Autodesk Inventor part; units mm, degrees
(part 3 of 3)
  arc A665 (615.7426, 1908.5354) -> (603.7426, 1896.5354) centre (615.7426, 1896.5354) ccw
  line L665 (643.2426, 1896.5354) -> (643.2426, 1908.5354)
  line L666 (36.3541, 1810.6764) -> (36.3541, 1843.6764)
  line L667 (311.3541, 1810.6764) -> (311.3541, 1843.6764)
  line L668 (311.3541, 1810.6764) -> (36.3541, 1810.6764)
  circle A666 centre (233.6541, 1827.1764) radius 3
  circle A667 centre (114.0541, 1827.1764) radius 3
  line L669 (36.3541, 1843.6764) -> (36.3541, 1855.6764)
  line L670 (311.3541, 1855.6764) -> (36.3541, 1855.6764)
  line L671 (311.3541, 1843.6764) -> (311.3541, 1855.6764)
  line L672 (594.2448, 1855.6764) -> (594.2448, 1843.6764)
  line L673 (319.2448, 1855.6764) -> (319.2448, 1843.6764)
  line L674 (319.2448, 1855.6764) -> (594.2448, 1855.6764)
  line L675 (594.2448, 1810.6764) -> (594.2448, 1843.6764)
  line L676 (319.2448, 1810.6764) -> (594.2448, 1810.6764)
  line L677 (319.2448, 1810.6764) -> (319.2448, 1843.6764)
  circle A668 centre (516.5448, 1827.1764) radius 3
  circle A669 centre (396.9448, 1827.1764) radius 3
  line L678 (791.8708, 1824.2966) -> (651.8708, 1824.2966)
  arc A670 (791.8708, 1824.2966) -> (801.8708, 1834.2966) centre (791.8708, 1834.2966) ccw
  line L679 (801.8708, 1834.2966) -> (801.8708, 1845.2966)
  line L680 (841.3708, 1845.2966) -> (841.3708, 1812.2966)
  line L681 (841.3708, 1812.2966) -> (602.3708, 1812.2966)
  line L682 (602.3708, 1845.2966) -> (602.3708, 1812.2966)
  arc A671 (641.8708, 1834.2966) -> (651.8708, 1824.2966) centre (651.8708, 1834.2966) ccw
  line L683 (641.8708, 1834.2966) -> (641.8708, 1845.2966)
  line L684 (829.3708, 1857.2966) -> (801.8708, 1857.2966)
  arc A672 (841.3708, 1845.2966) -> (829.3708, 1857.2966) centre (829.3708, 1845.2966) ccw
  line L685 (801.8708, 1845.2966) -> (801.8708, 1857.2966)
  line L686 (641.8708, 1857.2966) -> (614.3708, 1857.2966)
  arc A673 (614.3708, 1857.2966) -> (602.3708, 1845.2966) centre (614.3708, 1845.2966) ccw
  line L687 (641.8708, 1845.2966) -> (641.8708, 1857.2966)
  line L688 (312.2332, 1586.4479) -> (37.2332, 1586.4479)
  line L689 (312.2332, 1586.4479) -> (312.2332, 1801.4479)
  line L690 (37.2332, 1801.4479) -> (37.2332, 1586.4479)
  line L691 (312.2332, 1801.4479) -> (37.2332, 1801.4479)
  line L692 (594.0537, 1587.8293) -> (319.0537, 1587.8293)
  line L693 (594.0537, 1587.8293) -> (594.0537, 1802.8293)
  line L694 (319.0537, 1802.8293) -> (319.0537, 1587.8293)
  line L695 (594.0537, 1802.8293) -> (319.0537, 1802.8293)
  line L696 (879.1815, 1586.5894) -> (604.1815, 1586.5894)
  line L697 (879.1815, 1586.5894) -> (879.1815, 1801.5894)
  line L698 (604.1815, 1801.5894) -> (604.1815, 1586.5894)
  line L699 (879.1815, 1801.5894) -> (604.1815, 1801.5894)
  line L700 (35.4953, 1536.4526) -> (274.4953, 1536.4526)
  line L701 (35.4953, 1569.4526) -> (35.4953, 1536.4526)
  line L702 (274.4953, 1569.4526) -> (274.4953, 1536.4526)
  line L703 (47.4953, 1581.4526) -> (262.4953, 1581.4526)
  arc A674 (274.4953, 1569.4526) -> (262.4953, 1581.4526) centre (262.4953, 1569.4526) ccw
  arc A675 (47.4953, 1581.4526) -> (35.4953, 1569.4526) centre (47.4953, 1569.4526) ccw
  line L704 (280.016, 1536.4526) -> (519.016, 1536.4526)
  line L705 (280.016, 1569.4526) -> (280.016, 1536.4526)
  line L706 (519.016, 1569.4526) -> (519.016, 1536.4526)
  line L707 (292.016, 1581.4526) -> (507.016, 1581.4526)
  arc A676 (519.016, 1569.4526) -> (507.016, 1581.4526) centre (507.016, 1569.4526) ccw
  arc A677 (292.016, 1581.4526) -> (280.016, 1569.4526) centre (292.016, 1569.4526) ccw
  line L708 (523.243, 1536.8823) -> (762.243, 1536.8823)
  line L709 (523.243, 1569.8823) -> (523.243, 1536.8823)
  line L710 (762.243, 1569.8823) -> (762.243, 1536.8823)
  line L711 (535.243, 1581.8823) -> (750.243, 1581.8823)
  arc A678 (762.243, 1569.8823) -> (750.243, 1581.8823) centre (750.243, 1569.8823) ccw
  arc A679 (535.243, 1581.8823) -> (523.243, 1569.8823) centre (535.243, 1569.8823) ccw
  circle A680 centre (711.5153, 1953.9544) radius 3
  circle A681 centre (651.7153, 1953.9544) radius 3
  arc A682 (711.5153, 1948.9544) -> (711.5153, 1958.9544) centre (711.5153, 1953.9544) ccw
  line L712 (711.5153, 1948.9544) -> (651.7153, 1948.9544)
  arc A683 (651.7153, 1958.9544) -> (651.7153, 1948.9544) centre (651.7153, 1953.9544) ccw
  line L713 (711.5153, 1958.9544) -> (651.7153, 1958.9544)
  circle A684 centre (786.612, 1954.088) radius 3
  circle A685 centre (726.812, 1954.088) radius 3
  arc A686 (786.612, 1949.088) -> (786.612, 1959.088) centre (786.612, 1954.088) ccw
  line L714 (786.612, 1949.088) -> (726.812, 1949.088)
  arc A687 (726.812, 1959.088) -> (726.812, 1949.088) centre (726.812, 1954.088) ccw
  line L715 (786.612, 1959.088) -> (726.812, 1959.088)
  circle A688 centre (711.8432, 1938.9091) radius 3
  circle A689 centre (652.0432, 1938.9091) radius 3
  arc A690 (711.8432, 1933.9091) -> (711.8432, 1943.9091) centre (711.8432, 1938.9091) ccw
  line L716 (711.8432, 1933.9091) -> (652.0432, 1933.9091)
  arc A691 (652.0432, 1943.9091) -> (652.0432, 1933.9091) centre (652.0432, 1938.9091) ccw
  line L717 (711.8432, 1943.9091) -> (652.0432, 1943.9091)
  circle A692 centre (786.9399, 1939.0427) radius 3
  circle A693 centre (727.1399, 1939.0427) radius 3
  arc A694 (786.9399, 1934.0427) -> (786.9399, 1944.0427) centre (786.9399, 1939.0427) ccw
  line L718 (786.9399, 1934.0427) -> (727.1399, 1934.0427)
  arc A695 (727.1399, 1944.0427) -> (727.1399, 1934.0427) centre (727.1399, 1939.0427) ccw
  line L719 (786.9399, 1944.0427) -> (727.1399, 1944.0427)
  circle A696 centre (714.3507, 1902.6647) radius 3
  circle A697 centre (654.5507, 1902.6647) radius 3
  arc A698 (714.3507, 1897.6647) -> (714.3507, 1907.6647) centre (714.3507, 1902.6647) ccw
  line L720 (714.3507, 1897.6647) -> (654.5507, 1897.6647)
  arc A699 (654.5507, 1907.6647) -> (654.5507, 1897.6647) centre (654.5507, 1902.6647) ccw
  line L721 (714.3507, 1907.6647) -> (654.5507, 1907.6647)
  circle A700 centre (789.4474, 1902.7983) radius 3
  circle A701 centre (729.6474, 1902.7983) radius 3
  arc A702 (789.4474, 1897.7983) -> (789.4474, 1907.7983) centre (789.4474, 1902.7983) ccw
  line L722 (789.4474, 1897.7983) -> (729.6474, 1897.7983)
  arc A703 (729.6474, 1907.7983) -> (729.6474, 1897.7983) centre (729.6474, 1902.7983) ccw
  line L723 (789.4474, 1907.7983) -> (729.6474, 1907.7983)
  circle A704 centre (714.6786, 1887.6194) radius 3
  circle A705 centre (654.8786, 1887.6194) radius 3
  arc A706 (714.6786, 1882.6194) -> (714.6786, 1892.6194) centre (714.6786, 1887.6194) ccw
  line L724 (714.6786, 1882.6194) -> (654.8786, 1882.6194)
  arc A707 (654.8786, 1892.6194) -> (654.8786, 1882.6194) centre (654.8786, 1887.6194) ccw
  line L725 (714.6786, 1892.6194) -> (654.8786, 1892.6194)
  circle A708 centre (789.7753, 1887.7529) radius 3
  circle A709 centre (729.9753, 1887.7529) radius 3
  arc A710 (789.7753, 1882.7529) -> (789.7753, 1892.7529) centre (789.7753, 1887.7529) ccw
  line L726 (789.7753, 1882.7529) -> (729.9753, 1882.7529)
  arc A711 (729.9753, 1892.7529) -> (729.9753, 1882.7529) centre (729.9753, 1887.7529) ccw
  line L727 (789.7753, 1892.7529) -> (729.9753, 1892.7529)
  line L728 (35.9089, 1465.4839) -> (35.9089, 1498.4839)
  line L729 (310.9089, 1465.4839) -> (310.9089, 1498.4839)
  line L730 (310.9089, 1465.4839) -> (35.9089, 1465.4839)
  circle A712 centre (193.2089, 1492.9839) radius 3
  circle A713 centre (73.6089, 1492.9839) radius 3
  line L731 (35.9089, 1498.4839) -> (35.9089, 1510.4839)
  line L732 (310.9089, 1510.4839) -> (35.9089, 1510.4839)
  line L733 (310.9089, 1498.4839) -> (310.9089, 1510.4839)
  line L734 (789.1371, 1478.9516) -> (649.1371, 1478.9516)
  arc A714 (789.1371, 1478.9516) -> (799.1371, 1488.9516) centre (789.1371, 1488.9516) ccw
  line L735 (799.1371, 1488.9516) -> (799.1371, 1499.9516)
  line L736 (838.6371, 1499.9516) -> (838.6371, 1466.9516)
  line L737 (838.6371, 1466.9516) -> (599.6371, 1466.9516)
  line L738 (599.6371, 1499.9516) -> (599.6371, 1466.9516)
  arc A715 (639.1371, 1488.9516) -> (649.1371, 1478.9516) centre (649.1371, 1488.9516) ccw
  line L739 (639.1371, 1488.9516) -> (639.1371, 1499.9516)
  line L740 (826.6371, 1511.9516) -> (799.1371, 1511.9516)
  arc A716 (838.6371, 1499.9516) -> (826.6371, 1511.9516) centre (826.6371, 1499.9516) ccw
  line L741 (799.1371, 1499.9516) -> (799.1371, 1511.9516)
  line L742 (639.1371, 1511.9516) -> (611.6371, 1511.9516)
  arc A717 (611.6371, 1511.9516) -> (599.6371, 1499.9516) centre (611.6371, 1499.9516) ccw
  line L743 (639.1371, 1499.9516) -> (639.1371, 1511.9516)
  line L744 (310.5529, 1415.9284) -> (310.5529, 1448.9284)
  line L745 (35.5529, 1415.9284) -> (310.5529, 1415.9284)
  line L746 (35.5529, 1415.9284) -> (35.5529, 1448.9284)
  circle A718 centre (272.8529, 1432.4284) radius 3
  circle A719 centre (153.2529, 1432.4284) radius 3
  circle A720 centre (232.8529, 1443.4284) radius 3
  circle A721 centre (113.2529, 1443.4284) radius 3
  line L747 (310.5529, 1460.9284) -> (310.5529, 1448.9284)
  line L748 (35.5529, 1460.9284) -> (35.5529, 1448.9284)
  line L749 (35.5529, 1460.9284) -> (310.5529, 1460.9284)
  line L750 (592.7152, 1510.0135) -> (592.7152, 1498.0135)
  line L751 (317.7152, 1510.0135) -> (317.7152, 1498.0135)
  line L752 (317.7152, 1510.0135) -> (592.7152, 1510.0135)
  line L753 (592.7152, 1465.0135) -> (592.7152, 1498.0135)
  line L754 (317.7152, 1465.0135) -> (592.7152, 1465.0135)
  line L755 (317.7152, 1465.0135) -> (317.7152, 1498.0135)
  circle A722 centre (555.0152, 1492.5135) radius 3
  circle A723 centre (435.4152, 1492.5135) radius 3
  line L756 (317.5392, 1415.188) -> (317.5392, 1448.188)
  line L757 (592.5392, 1415.188) -> (592.5392, 1448.188)
  line L758 (592.5392, 1415.188) -> (317.5392, 1415.188)
  circle A724 centre (514.8392, 1442.688) radius 3
  circle A725 centre (395.2392, 1442.688) radius 3
  circle A726 centre (474.8392, 1431.688) radius 3
  circle A727 centre (355.2392, 1431.688) radius 3
  line L759 (317.5392, 1448.188) -> (317.5392, 1460.188)
  line L760 (592.5392, 1460.188) -> (317.5392, 1460.188)
  line L761 (592.5392, 1448.188) -> (592.5392, 1460.188)
  line L762 (791.6488, 1428.4028) -> (651.6488, 1428.4028)
  arc A728 (791.6488, 1428.4028) -> (801.6488, 1438.4028) centre (791.6488, 1438.4028) ccw
  line L763 (801.6488, 1438.4028) -> (801.6488, 1449.4028)
  line L764 (841.1488, 1449.4028) -> (841.1488, 1416.4028)
  line L765 (841.1488, 1416.4028) -> (602.1488, 1416.4028)
  line L766 (602.1488, 1449.4028) -> (602.1488, 1416.4028)
  arc A729 (641.6488, 1438.4028) -> (651.6488, 1428.4028) centre (651.6488, 1438.4028) ccw
  line L767 (641.6488, 1438.4028) -> (641.6488, 1449.4028)
  line L768 (829.1488, 1461.4028) -> (801.6488, 1461.4028)
  arc A730 (841.1488, 1449.4028) -> (829.1488, 1461.4028) centre (829.1488, 1449.4028) ccw
  line L769 (801.6488, 1449.4028) -> (801.6488, 1461.4028)
  line L770 (641.6488, 1461.4028) -> (614.1488, 1461.4028)
  arc A731 (614.1488, 1461.4028) -> (602.1488, 1449.4028) centre (614.1488, 1449.4028) ccw
  line L771 (641.6488, 1449.4028) -> (641.6488, 1461.4028)
  line L772 (34.7604, 1363.5438) -> (34.7604, 1396.5438)
  line L773 (309.7604, 1363.5438) -> (309.7604, 1396.5438)
  line L774 (309.7604, 1363.5438) -> (34.7604, 1363.5438)
  circle A732 centre (232.0604, 1380.0438) radius 3
  circle A733 centre (112.4604, 1380.0438) radius 3
  line L775 (34.7604, 1396.5438) -> (34.7604, 1408.5438)
  line L776 (309.7604, 1408.5438) -> (34.7604, 1408.5438)
  line L777 (309.7604, 1396.5438) -> (309.7604, 1408.5438)
  line L778 (592.6511, 1408.5438) -> (592.6511, 1396.5438)
  line L779 (317.6511, 1408.5438) -> (317.6511, 1396.5438)
  line L780 (317.6511, 1408.5438) -> (592.6511, 1408.5438)
  line L781 (592.6511, 1363.5438) -> (592.6511, 1396.5438)
  line L782 (317.6511, 1363.5438) -> (592.6511, 1363.5438)
  line L783 (317.6511, 1363.5438) -> (317.6511, 1396.5438)
  circle A734 centre (514.9511, 1380.0438) radius 3
  circle A735 centre (395.3511, 1380.0438) radius 3
  line L784 (790.277, 1377.164) -> (650.277, 1377.164)
  arc A736 (790.277, 1377.164) -> (800.277, 1387.164) centre (790.277, 1387.164) ccw
  line L785 (800.277, 1387.164) -> (800.277, 1398.164)
  line L786 (839.777, 1398.164) -> (839.777, 1365.164)
  line L787 (839.777, 1365.164) -> (600.777, 1365.164)
  line L788 (600.777, 1398.164) -> (600.777, 1365.164)
  arc A737 (640.277, 1387.164) -> (650.277, 1377.164) centre (650.277, 1387.164) ccw
  line L789 (640.277, 1387.164) -> (640.277, 1398.164)
  line L790 (827.777, 1410.164) -> (800.277, 1410.164)
  arc A738 (839.777, 1398.164) -> (827.777, 1410.164) centre (827.777, 1398.164) ccw
  line L791 (800.277, 1398.164) -> (800.277, 1410.164)
  line L792 (640.277, 1410.164) -> (612.777, 1410.164)
  arc A739 (612.777, 1410.164) -> (600.777, 1398.164) centre (612.777, 1398.164) ccw
  line L793 (640.277, 1398.164) -> (640.277, 1410.164)
  line L794 (310.6395, 1139.3153) -> (35.6395, 1139.3153)
  line L795 (310.6395, 1139.3153) -> (310.6395, 1354.3153)
  line L796 (35.6395, 1354.3153) -> (35.6395, 1139.3153)
  line L797 (310.6395, 1354.3153) -> (35.6395, 1354.3153)
  line L798 (592.4599, 1140.6967) -> (317.4599, 1140.6967)
  line L799 (592.4599, 1140.6967) -> (592.4599, 1355.6967)
  line L800 (317.4599, 1355.6967) -> (317.4599, 1140.6967)
  line L801 (592.4599, 1355.6967) -> (317.4599, 1355.6967)
  line L802 (877.5877, 1139.4569) -> (602.5877, 1139.4569)
  line L803 (877.5877, 1139.4569) -> (877.5877, 1354.4569)
  line L804 (602.5877, 1354.4569) -> (602.5877, 1139.4569)
  line L805 (877.5877, 1354.4569) -> (602.5877, 1354.4569)
  line L806 (33.9015, 1089.32) -> (272.9015, 1089.32)
  line L807 (33.9015, 1122.32) -> (33.9015, 1089.32)
  line L808 (272.9015, 1122.32) -> (272.9015, 1089.32)
  line L809 (45.9015, 1134.32) -> (260.9015, 1134.32)
  arc A740 (272.9015, 1122.32) -> (260.9015, 1134.32) centre (260.9015, 1122.32) ccw
  arc A741 (45.9015, 1134.32) -> (33.9015, 1122.32) centre (45.9015, 1122.32) ccw
  line L810 (278.4222, 1089.32) -> (517.4222, 1089.32)
  line L811 (278.4222, 1122.32) -> (278.4222, 1089.32)
  line L812 (517.4222, 1122.32) -> (517.4222, 1089.32)
  line L813 (290.4222, 1134.32) -> (505.4222, 1134.32)
  arc A742 (517.4222, 1122.32) -> (505.4222, 1134.32) centre (505.4222, 1122.32) ccw
  arc A743 (290.4222, 1134.32) -> (278.4222, 1122.32) centre (290.4222, 1122.32) ccw
  line L814 (521.6493, 1089.7497) -> (760.6493, 1089.7497)
  line L815 (521.6493, 1122.7497) -> (521.6493, 1089.7497)
  line L816 (760.6493, 1122.7497) -> (760.6493, 1089.7497)
  line L817 (533.6493, 1134.7497) -> (748.6493, 1134.7497)
  arc A744 (760.6493, 1122.7497) -> (748.6493, 1134.7497) centre (748.6493, 1122.7497) ccw
  arc A745 (533.6493, 1134.7497) -> (521.6493, 1122.7497) centre (533.6493, 1122.7497) ccw
  circle A746 centre (709.9216, 1506.8218) radius 3
  circle A747 centre (650.1216, 1506.8218) radius 3
  arc A748 (709.9216, 1501.8218) -> (709.9216, 1511.8218) centre (709.9216, 1506.8218) ccw
  line L818 (709.9216, 1501.8218) -> (650.1216, 1501.8218)
  arc A749 (650.1216, 1511.8218) -> (650.1216, 1501.8218) centre (650.1216, 1506.8218) ccw
  line L819 (709.9216, 1511.8218) -> (650.1216, 1511.8218)
  circle A750 centre (785.0182, 1506.9554) radius 3
  circle A751 centre (725.2182, 1506.9554) radius 3
  arc A752 (785.0182, 1501.9554) -> (785.0182, 1511.9554) centre (785.0182, 1506.9554) ccw
  line L820 (785.0182, 1501.9554) -> (725.2182, 1501.9554)
  arc A753 (725.2182, 1511.9554) -> (725.2182, 1501.9554) centre (725.2182, 1506.9554) ccw
  line L821 (785.0182, 1511.9554) -> (725.2182, 1511.9554)
  circle A754 centre (710.2495, 1491.7765) radius 3
  circle A755 centre (650.4495, 1491.7765) radius 3
  arc A756 (710.2495, 1486.7765) -> (710.2495, 1496.7765) centre (710.2495, 1491.7765) ccw
  line L822 (710.2495, 1486.7765) -> (650.4495, 1486.7765)
  arc A757 (650.4495, 1496.7765) -> (650.4495, 1486.7765) centre (650.4495, 1491.7765) ccw
  line L823 (710.2495, 1496.7765) -> (650.4495, 1496.7765)
  circle A758 centre (785.3462, 1491.9101) radius 3
  circle A759 centre (725.5462, 1491.9101) radius 3
  arc A760 (785.3462, 1486.9101) -> (785.3462, 1496.9101) centre (785.3462, 1491.9101) ccw
  line L824 (785.3462, 1486.9101) -> (725.5462, 1486.9101)
  arc A761 (725.5462, 1496.9101) -> (725.5462, 1486.9101) centre (725.5462, 1491.9101) ccw
  line L825 (785.3462, 1496.9101) -> (725.5462, 1496.9101)
  circle A762 centre (712.757, 1455.5321) radius 3
  circle A763 centre (652.957, 1455.5321) radius 3
  arc A764 (712.757, 1450.5321) -> (712.757, 1460.5321) centre (712.757, 1455.5321) ccw
  line L826 (712.757, 1450.5321) -> (652.957, 1450.5321)
  arc A765 (652.957, 1460.5321) -> (652.957, 1450.5321) centre (652.957, 1455.5321) ccw
  line L827 (712.757, 1460.5321) -> (652.957, 1460.5321)
  circle A766 centre (787.8536, 1455.6657) radius 3
  circle A767 centre (728.0536, 1455.6657) radius 3
  arc A768 (787.8536, 1450.6657) -> (787.8536, 1460.6657) centre (787.8536, 1455.6657) ccw
  line L828 (787.8536, 1450.6657) -> (728.0536, 1450.6657)
  arc A769 (728.0536, 1460.6657) -> (728.0536, 1450.6657) centre (728.0536, 1455.6657) ccw
  line L829 (787.8536, 1460.6657) -> (728.0536, 1460.6657)
  circle A770 centre (713.0849, 1440.4868) radius 3
  circle A771 centre (653.2849, 1440.4868) radius 3
  arc A772 (713.0849, 1435.4868) -> (713.0849, 1445.4868) centre (713.0849, 1440.4868) ccw
  line L830 (713.0849, 1435.4868) -> (653.2849, 1435.4868)
  arc A773 (653.2849, 1445.4868) -> (653.2849, 1435.4868) centre (653.2849, 1440.4868) ccw
  line L831 (713.0849, 1445.4868) -> (653.2849, 1445.4868)
  circle A774 centre (788.1816, 1440.6204) radius 3
  circle A775 centre (728.3816, 1440.6204) radius 3
  arc A776 (788.1816, 1435.6204) -> (788.1816, 1445.6204) centre (788.1816, 1440.6204) ccw
  line L832 (788.1816, 1435.6204) -> (728.3816, 1435.6204)
  arc A777 (728.3816, 1445.6204) -> (728.3816, 1435.6204) centre (728.3816, 1440.6204) ccw
  line L833 (788.1816, 1445.6204) -> (728.3816, 1445.6204)
  line L834 (24.9276, 1026.8577) -> (24.9276, 1059.8577)
  line L835 (299.9276, 1026.8577) -> (299.9276, 1059.8577)
  line L836 (299.9276, 1026.8577) -> (24.9276, 1026.8577)
  circle A778 centre (182.2276, 1054.3577) radius 3
  circle A779 centre (62.6276, 1054.3577) radius 3
  line L837 (24.9276, 1059.8577) -> (24.9276, 1071.8577)
  line L838 (299.9276, 1071.8577) -> (24.9276, 1071.8577)
  line L839 (299.9276, 1059.8577) -> (299.9276, 1071.8577)
  line L840 (778.1558, 1040.3254) -> (638.1558, 1040.3254)
  arc A780 (778.1558, 1040.3254) -> (788.1558, 1050.3254) centre (778.1558, 1050.3254) ccw
  line L841 (788.1558, 1050.3254) -> (788.1558, 1061.3254)
  line L842 (827.6558, 1061.3254) -> (827.6558, 1028.3254)
  line L843 (827.6558, 1028.3254) -> (588.6558, 1028.3254)
  line L844 (588.6558, 1061.3254) -> (588.6558, 1028.3254)
  arc A781 (628.1558, 1050.3254) -> (638.1558, 1040.3254) centre (638.1558, 1050.3254) ccw
  line L845 (628.1558, 1050.3254) -> (628.1558, 1061.3254)
  line L846 (815.6558, 1073.3254) -> (788.1558, 1073.3254)
  arc A782 (827.6558, 1061.3254) -> (815.6558, 1073.3254) centre (815.6558, 1061.3254) ccw
  line L847 (788.1558, 1061.3254) -> (788.1558, 1073.3254)
  line L848 (628.1558, 1073.3254) -> (600.6558, 1073.3254)
  arc A783 (600.6558, 1073.3254) -> (588.6558, 1061.3254) centre (600.6558, 1061.3254) ccw
  line L849 (628.1558, 1061.3254) -> (628.1558, 1073.3254)
  line L850 (299.5716, 977.3022) -> (299.5716, 1010.3022)
  line L851 (24.5716, 977.3022) -> (299.5716, 977.3022)
  line L852 (24.5716, 977.3022) -> (24.5716, 1010.3022)
  circle A784 centre (261.8716, 993.8022) radius 3
  circle A785 centre (142.2716, 993.8022) radius 3
  circle A786 centre (221.8716, 1004.8022) radius 3
  circle A787 centre (102.2716, 1004.8022) radius 3
  line L853 (299.5716, 1022.3022) -> (299.5716, 1010.3022)
  line L854 (24.5716, 1022.3022) -> (24.5716, 1010.3022)
  line L855 (24.5716, 1022.3022) -> (299.5716, 1022.3022)
  line L856 (581.7339, 1071.3873) -> (581.7339, 1059.3873)
  line L857 (306.7339, 1071.3873) -> (306.7339, 1059.3873)
  line L858 (306.7339, 1071.3873) -> (581.7339, 1071.3873)
  line L859 (581.7339, 1026.3873) -> (581.7339, 1059.3873)
  line L860 (306.7339, 1026.3873) -> (581.7339, 1026.3873)
  line L861 (306.7339, 1026.3873) -> (306.7339, 1059.3873)
  circle A788 centre (544.0339, 1053.8873) radius 3
  circle A789 centre (424.4339, 1053.8873) radius 3
  line L862 (306.5579, 976.5618) -> (306.5579, 1009.5618)
  line L863 (581.5579, 976.5618) -> (581.5579, 1009.5618)
  line L864 (581.5579, 976.5618) -> (306.5579, 976.5618)
  circle A790 centre (503.8579, 1004.0618) radius 3
  circle A791 centre (384.2579, 1004.0618) radius 3
  circle A792 centre (463.8579, 993.0618) radius 3
  circle A793 centre (344.2579, 993.0618) radius 3
  line L865 (306.5579, 1009.5618) -> (306.5579, 1021.5618)
  line L866 (581.5579, 1021.5618) -> (306.5579, 1021.5618)
  line L867 (581.5579, 1009.5618) -> (581.5579, 1021.5618)
  line L868 (780.6675, 989.7766) -> (640.6675, 989.7766)
  arc A794 (780.6675, 989.7766) -> (790.6675, 999.7766) centre (780.6675, 999.7766) ccw
  line L869 (790.6675, 999.7766) -> (790.6675, 1010.7766)
  line L870 (830.1675, 1010.7766) -> (830.1675, 977.7766)
  line L871 (830.1675, 977.7766) -> (591.1675, 977.7766)
  line L872 (591.1675, 1010.7766) -> (591.1675, 977.7766)
  arc A795 (630.6675, 999.7766) -> (640.6675, 989.7766) centre (640.6675, 999.7766) ccw
  line L873 (630.6675, 999.7766) -> (630.6675, 1010.7766)
  line L874 (818.1675, 1022.7766) -> (790.6675, 1022.7766)
  arc A796 (830.1675, 1010.7766) -> (818.1675, 1022.7766) centre (818.1675, 1010.7766) ccw
  line L875 (790.6675, 1010.7766) -> (790.6675, 1022.7766)
  line L876 (630.6675, 1022.7766) -> (603.1675, 1022.7766)
  arc A797 (603.1675, 1022.7766) -> (591.1675, 1010.7766) centre (603.1675, 1010.7766) ccw
  line L877 (630.6675, 1010.7766) -> (630.6675, 1022.7766)
  line L878 (23.7791, 924.9176) -> (23.7791, 957.9176)
  line L879 (298.7791, 924.9176) -> (298.7791, 957.9176)
  line L880 (298.7791, 924.9176) -> (23.7791, 924.9176)
  circle A798 centre (221.0791, 941.4176) radius 3
  circle A799 centre (101.4791, 941.4176) radius 3
  line L881 (23.7791, 957.9176) -> (23.7791, 969.9176)
  line L882 (298.7791, 969.9176) -> (23.7791, 969.9176)
  line L883 (298.7791, 957.9176) -> (298.7791, 969.9176)
  line L884 (581.6698, 969.9176) -> (581.6698, 957.9176)
  line L885 (306.6698, 969.9176) -> (306.6698, 957.9176)
  line L886 (306.6698, 969.9176) -> (581.6698, 969.9176)
  line L887 (581.6698, 924.9176) -> (581.6698, 957.9176)
  line L888 (306.6698, 924.9176) -> (581.6698, 924.9176)
  line L889 (306.6698, 924.9176) -> (306.6698, 957.9176)
  circle A800 centre (503.9698, 941.4176) radius 3
  circle A801 centre (384.3698, 941.4176) radius 3
  line L890 (779.2957, 938.5378) -> (639.2957, 938.5378)
  arc A802 (779.2957, 938.5378) -> (789.2957, 948.5378) centre (779.2957, 948.5378) ccw
  line L891 (789.2957, 948.5378) -> (789.2957, 959.5378)
  line L892 (828.7957, 959.5378) -> (828.7957, 926.5378)
  line L893 (828.7957, 926.5378) -> (589.7957, 926.5378)
  line L894 (589.7957, 959.5378) -> (589.7957, 926.5378)
  arc A803 (629.2957, 948.5378) -> (639.2957, 938.5378) centre (639.2957, 948.5378) ccw
  line L895 (629.2957, 948.5378) -> (629.2957, 959.5378)
  line L896 (816.7957, 971.5378) -> (789.2957, 971.5378)
  arc A804 (828.7957, 959.5378) -> (816.7957, 971.5378) centre (816.7957, 959.5378) ccw
  line L897 (789.2957, 959.5378) -> (789.2957, 971.5378)
  line L898 (629.2957, 971.5378) -> (601.7957, 971.5378)
  arc A805 (601.7957, 971.5378) -> (589.7957, 959.5378) centre (601.7957, 959.5378) ccw
  line L899 (629.2957, 959.5378) -> (629.2957, 971.5378)
  line L900 (299.6582, 700.6891) -> (24.6582, 700.6891)
  line L901 (299.6582, 700.6891) -> (299.6582, 915.6891)
  line L902 (24.6582, 915.6891) -> (24.6582, 700.6891)
  line L903 (299.6582, 915.6891) -> (24.6582, 915.6891)
  line L904 (581.4786, 702.0706) -> (306.4786, 702.0706)
  line L905 (581.4786, 702.0706) -> (581.4786, 917.0706)
  line L906 (306.4786, 917.0706) -> (306.4786, 702.0706)
  line L907 (581.4786, 917.0706) -> (306.4786, 917.0706)
  line L908 (866.6064, 700.8307) -> (591.6064, 700.8307)
  line L909 (866.6064, 700.8307) -> (866.6064, 915.8307)
  line L910 (591.6064, 915.8307) -> (591.6064, 700.8307)
  line L911 (866.6064, 915.8307) -> (591.6064, 915.8307)
  line L912 (22.9202, 650.6939) -> (261.9202, 650.6939)
  line L913 (22.9202, 683.6939) -> (22.9202, 650.6939)
  line L914 (261.9202, 683.6939) -> (261.9202, 650.6939)
  line L915 (34.9202, 695.6939) -> (249.9202, 695.6939)
  arc A806 (261.9202, 683.6939) -> (249.9202, 695.6939) centre (249.9202, 683.6939) ccw
  arc A807 (34.9202, 695.6939) -> (22.9202, 683.6939) centre (34.9202, 683.6939) ccw
  line L916 (267.4409, 650.6939) -> (506.4409, 650.6939)
  line L917 (267.4409, 683.6939) -> (267.4409, 650.6939)
  line L918 (506.4409, 683.6939) -> (506.4409, 650.6939)
  line L919 (279.4409, 695.6939) -> (494.4409, 695.6939)
  arc A808 (506.4409, 683.6939) -> (494.4409, 695.6939) centre (494.4409, 683.6939) ccw
  arc A809 (279.4409, 695.6939) -> (267.4409, 683.6939) centre (279.4409, 683.6939) ccw
  line L920 (510.668, 651.1235) -> (749.668, 651.1235)
  line L921 (510.668, 684.1235) -> (510.668, 651.1235)
  line L922 (749.668, 684.1235) -> (749.668, 651.1235)
  line L923 (522.668, 696.1235) -> (737.668, 696.1235)
  arc A810 (749.668, 684.1235) -> (737.668, 696.1235) centre (737.668, 684.1235) ccw
  arc A811 (522.668, 696.1235) -> (510.668, 684.1235) centre (522.668, 684.1235) ccw
  circle A812 centre (698.9403, 1068.1956) radius 3
  circle A813 centre (639.1403, 1068.1956) radius 3
  arc A814 (698.9403, 1063.1956) -> (698.9403, 1073.1956) centre (698.9403, 1068.1956) ccw
  line L924 (698.9403, 1063.1956) -> (639.1403, 1063.1956)
  arc A815 (639.1403, 1073.1956) -> (639.1403, 1063.1956) centre (639.1403, 1068.1956) ccw
  line L925 (698.9403, 1073.1956) -> (639.1403, 1073.1956)
  circle A816 centre (774.0369, 1068.3292) radius 3
  circle A817 centre (714.2369, 1068.3292) radius 3
  arc A818 (774.0369, 1063.3292) -> (774.0369, 1073.3292) centre (774.0369, 1068.3292) ccw
  line L926 (774.0369, 1063.3292) -> (714.2369, 1063.3292)
  arc A819 (714.2369, 1073.3292) -> (714.2369, 1063.3292) centre (714.2369, 1068.3292) ccw
  line L927 (774.0369, 1073.3292) -> (714.2369, 1073.3292)
  circle A820 centre (699.2682, 1053.1503) radius 3
  circle A821 centre (639.4682, 1053.1503) radius 3
  arc A822 (699.2682, 1048.1503) -> (699.2682, 1058.1503) centre (699.2682, 1053.1503) ccw
  line L928 (699.2682, 1048.1503) -> (639.4682, 1048.1503)
  arc A823 (639.4682, 1058.1503) -> (639.4682, 1048.1503) centre (639.4682, 1053.1503) ccw
  line L929 (699.2682, 1058.1503) -> (639.4682, 1058.1503)
  circle A824 centre (774.3649, 1053.2839) radius 3
  circle A825 centre (714.5649, 1053.2839) radius 3
  arc A826 (774.3649, 1048.2839) -> (774.3649, 1058.2839) centre (774.3649, 1053.2839) ccw
  line L930 (774.3649, 1048.2839) -> (714.5649, 1048.2839)
  arc A827 (714.5649, 1058.2839) -> (714.5649, 1048.2839) centre (714.5649, 1053.2839) ccw
  line L931 (774.3649, 1058.2839) -> (714.5649, 1058.2839)
  circle A828 centre (701.7757, 1016.9059) radius 3
  circle A829 centre (641.9757, 1016.9059) radius 3
  arc A830 (701.7757, 1011.9059) -> (701.7757, 1021.9059) centre (701.7757, 1016.9059) ccw
  line L932 (701.7757, 1011.9059) -> (641.9757, 1011.9059)
  arc A831 (641.9757, 1021.9059) -> (641.9757, 1011.9059) centre (641.9757, 1016.9059) ccw
  line L933 (701.7757, 1021.9059) -> (641.9757, 1021.9059)
  circle A832 centre (776.8723, 1017.0395) radius 3
  circle A833 centre (717.0723, 1017.0395) radius 3
  arc A834 (776.8723, 1012.0395) -> (776.8723, 1022.0395) centre (776.8723, 1017.0395) ccw
  line L934 (776.8723, 1012.0395) -> (717.0723, 1012.0395)
  arc A835 (717.0723, 1022.0395) -> (717.0723, 1012.0395) centre (717.0723, 1017.0395) ccw
  line L935 (776.8723, 1022.0395) -> (717.0723, 1022.0395)
  circle A836 centre (702.1036, 1001.8606) radius 3
  circle A837 centre (642.3036, 1001.8606) radius 3
  arc A838 (702.1036, 996.8606) -> (702.1036, 1006.8606) centre (702.1036, 1001.8606) ccw
  line L936 (702.1036, 996.8606) -> (642.3036, 996.8606)
  arc A839 (642.3036, 1006.8606) -> (642.3036, 996.8606) centre (642.3036, 1001.8606) ccw
  line L937 (702.1036, 1006.8606) -> (642.3036, 1006.8606)
  circle A840 centre (777.2003, 1001.9942) radius 3
  circle A841 centre (717.4003, 1001.9942) radius 3
  arc A842 (777.2003, 996.9942) -> (777.2003, 1006.9942) centre (777.2003, 1001.9942) ccw
  line L938 (777.2003, 996.9942) -> (717.4003, 996.9942)
  arc A843 (717.4003, 1006.9942) -> (717.4003, 996.9942) centre (717.4003, 1001.9942) ccw
  line L939 (777.2003, 1006.9942) -> (717.4003, 1006.9942)
  line L940 (0, 0) -> (1850, 0)
  line L941 (1850, 0) -> (1850, 2440)
  line L942 (1850, 2440) -> (0, 2440)
  line L943 (0, 2440) -> (0, 0)
  line L944 (1007.0665, 2314.7275) -> (1085.5401, 2314.7275) construction
  line L945 (1085.5401, 2314.7275) -> (1085.5401, 2300.5013) construction
  line L946 (1085.5401, 2300.5013) -> (1007.0665, 2300.5013) construction
  line L947 (1007.0665, 2300.5013) -> (1007.0665, 2314.7275) construction
  point P0 (904.9656, 2168.2558)
  point P1 (1194.1078, 2168.2558)
  point P2 (1194.1078, 2249.7064)
  point P3 (904.9656, 2249.7064)
  point P4 (929.5367, 2208.9811)
  point P5 (979.697, 2161.6606)
  point P6 (981.0367, 2166.6606)
  point P7 (981.0367, 2251.3016)
  point P8 (979.697, 2256.3016)
  point P9 (961.2527, 2288.248)
  point P10 (995.697, 2256.3016)
  point P11 (997.0367, 2251.3016)
  point P12 (997.0367, 2166.6606)
  point P13 (995.697, 2161.6606)
  point P14 (1125.8207, 2295.1762)
  point P15 (1532.6771, 2116.2231)
  point P16 (1447.2348, 2220.4015)
  point P17 (1253.0938, 2091.2231)
  point P18 (1283.1771, 2143.3289)
  point P19 (1430.0105, 2172.611)
  point P20 (1224.2874, 2235.8325)
  point P21 (1296.9285, 2111.2385)
  point P22 (1290.9657, 2114.6956)
  point P23 (1288.5063, 2110.8656)
  point P24 (1306.7616, 2118.8636)
  point P25 (1304.9194, 2110.2861)
  point P26 (1296.9285, 2095.0314)
  point P27 (1303.9736, 2396.0804)
  point P28 (1275.9561, 2398.137)
  point P29 (1267.7664, 2388.1171)
  point P30 (1445.2481, 2392.7629)
  point P31 (1017.3509, 2407.1763)
  point P32 (1182.3115, 2355.22)
  dimension "d0" = 1850
  dimension "d1" = 2440
  constraints: 1664 end point, 1152 point on circle, 844 centre point, 2 parallel, 1 horizontal, 1 perpendicular, 74 other
  measures "d0" distance of L942.end L941.end
  measures "d1" distance of L941.end L940.end
extrude "Extrusión1" add sketch "Visible" along normal blind 12 contours L128 A96 L129 A97 S2 S3 A98 L134 A99 L135 A100 L117 A101 S0 S1 A102 L127 A95
extrude "Extrusión2" add sketch "Visible" along normal blind 12 separate body contours L148 A118 L149 A119 L150 A120 L151 A121 L141 A122 L142 A123 L143 L144 L145 A124 L146 A125 L147 A117
extrude "Extrusión3" add sketch "Visible" along normal blind 12 separate body contours A128 A129 L152 A130 L153 A131 L154 A132 L155 A133 L156 A134 L157 A135 L158 A136 L159 A137 L160 A138 L161 A139 L162 A140 L163
extrude "Extrusión4" add sketch "Visible" along normal blind 12 separate body contours L101 L102 A63 L103 A64 L104
extrude "Extrusión5" add sketch "Visible" along normal blind 12 separate body contours L94 L95 L96 L93
extrude "Extrusión6" add sketch "Visible" along normal blind 12 separate body contours L98 L99 L100 L97
extrude "Extrusión7" add sketch "Visible" along normal blind 12 separate body contours A515 A516 L541 A517 L542 A518 L543 A519 L544 A520 L545 A521 L546 A522 L547 A523 L548 A524 L549 A525 L550 A526 L551 A527 L552
extrude "Extrusión8" add sketch "Visible" along normal blind 12 separate body contours A533 A534 L553 A538 A537 A535 L554 A532
extrude "Extrusión9" add sketch "Visible" along normal blind 12 separate body contours A85 A86 L113 A90 A89 A87 L114 A84
extrude "Extrusión10" add sketch "Visible" along normal blind 12 separate body contours A168 L203 A171 L201 A170 L202 A169 L200
extrude "Extrusión11" add sketch "Visible" along normal blind 12 separate body contours L168 A155 L174 A164 L171 A163 L173 A159 L176 A165 L178 A167 L179 A166 L172 A160 L175 A158 L170 A162 L177 A156 L169 A154 A152
extrude "Extrusión12" add sketch "Visible" along normal blind 12 separate body contours A151 L167 A149 L165 A148 L166 A150 L164
extrude "Extrusión13" add sketch "Visible" along normal blind 12 separate body contours A181 L207 A179 L205 A178 L206 A180 L204
